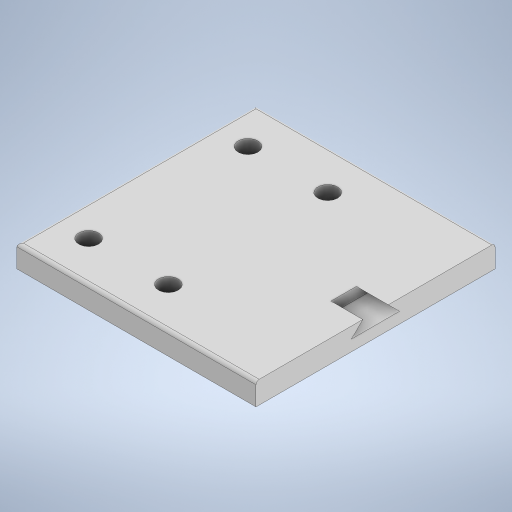
# Autodesk Inventor part: Dovetail_holder_V3
Saved by Autodesk Inventor 2023.2 (Build 272271000, 271)
## iProperties
Created: 2020-11-04
Part Number: Dovetail_holder_V3
Material: Generic
Document SubType Name: Modeling
Designer: Allesfresser
Density: 1 g/cm^3
Appearance: Default
Author: Allesfresser
Autodesk Inventor part; units mm, degrees
ref_plane "YZ Plane" through (0, 0, 0) normal (1, 0, 0) x (0, 1, 0)
ref_plane "XZ Plane" through (0, 0, 0) normal (0, 1, 0) x (-1, 0, 0)
ref_plane "XY Plane" through (0, 0, 0) normal (0, 0, 1) x (1, 0, 0)
sketch "Sketch1" plane through (0, 0, 0) normal (0, 1, 0) x (-1, 0, 0)
  line L0 (-37.5, 37.5) -> (37.5, 37.5)
  line L1 (37.5, 37.5) -> (37.5, -37.5)
  line L2 (37.5, -37.5) -> (-37.5, -37.5)
  line L3 (-37.5, -37.5) -> (-37.5, 37.5)
  line L4 (-37.5, 37.5) -> (37.5, -37.5) construction
  line L5 (37.5, 37.5) -> (-37.5, -37.5) construction
  point P0 (0, 0)
  dimension "d0" = 75
  dimension "d1" = 75
  constraints: 12 end point, 2 midpoint, 2 parallel, 1 horizontal, 1 perpendicular
  measures "d0" distance of L1.end L2.end
  measures "d1" distance of L0.end L1.end
extrude "Extrusion1" add sketch "Sketch1" along normal blind 7
sketch "Sketch2" plane through (0, 7, 0) normal (0, 1, 0) x (1, 0, 0)
  circle A0 centre (-27.5, -25) radius 3.1
  line L0 (-37.5, -37.5) -> (37.5, -37.5) projected
  line L1 (37.5, -37.5) -> (37.5, 37.5) projected
  circle A1 centre (-2.5, -25) radius 3.1
  point P0 (0, 0)
  dimension "d4" = 6.2
  dimension "d5" = 12.5
  dimension "d6" = 65
  dimension "d19" = 6.2
  dimension "d20" = 12.5
  dimension "d21" = 40
  constraints: 2 centre point
  measures "d4" diameter of A0
  measures "d5" distance from line of L0 A0.centre
  measures "d6" distance from line of L1 A0.centre
  measures "d19" diameter of A1
  measures "d20" distance from line of L0 A1.centre
  measures "d21" distance from line of L1 A1.centre
extrude "Extrusion2" cut sketch "Sketch2" against normal through all
mirror "Mirror1" about plane through (0, 0, 0) normal (0, 0, 1) of "Extrusion2"
sketch "Sketch3" plane through (37.5, 0, 37.5) normal (1, 0, 0) x (0, 0, -1)
  line L0 (0, 7) -> (75, 7) projected
  line L1 (33.5, 7) -> (29.9645, 3.4645)
  line L2 (33.5, 7) -> (38.5, 7) construction
  line L3 (33.5, 7) -> (41.5, 7)
  line L4 (33.5, 7) -> (41.5, 7) construction
  line L5 (41.5, 7) -> (45.0355, 3.4645)
  line L6 (45.0355, 3.4645) -> (29.9645, 3.4645)
  point P0 (37.5, 0)
  dimension "d9" = 5
  dimension "d10" = 135
  dimension "d11" = 33.5
  dimension "d12" = 8
  dimension "d13" = 0
  dimension "d14" = 5
  dimension "d15" = 135
  constraints: 12 end point, 2 equal length, 2 horizontal, 2 point on line, 1 collinear, 1 parallel
  measures "d9" distance of L1.start L1.end
  measures "d10" angle of L1 L2
  measures "d11" distance of L0.start L1.start
  measures "d12" distance of L1.start L3.end
  measures "d13" distance between parallel lines of L3 L4
  measures "d14" distance of L3.end L5.end
  measures "d15" angle of L3 L5
extrude "Extrusion3" cut sketch "Sketch3" against normal blind 10
fillet "Fillet1" radius 1 3 edges at (0, 7, -37.5) (-37.5, 7, 0) (0, 7, 37.5)
body "Solid1"
